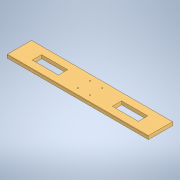
# Autodesk Inventor part: VerstaerkungHintenMitte
Saved by Autodesk Inventor 2020.3 (Build 243373010, 373A)
## iProperties
Created: 2021-02-13
Part Number: VerstaerkungHintenMitte
Material: Generisch
Document SubType Name: Modeling
Designer: Stefan
Density: 1 g/cm^3
Appearance: Fichte
Author: Stefan
Autodesk Inventor part; units mm, degrees
ref_plane "YZ Plane" through (0, 0, 0) normal (1, 0, 0) x (0, 1, 0)
ref_plane "XZ Plane" through (0, 0, 0) normal (0, 1, 0) x (-1, 0, 0)
ref_plane "XY Plane" through (0, 0, 0) normal (0, 0, 1) x (1, 0, 0)
sketch "Skizze1" plane through (0, 0, 0) normal (0, 1, 0) x (-1, 0, 0)
  line L0 (625.4144, 33.4967) -> (-184.5856, 33.4967)
  line L1 (-184.5856, 33.4967) -> (-184.5856, -108.5033)
  line L2 (-184.5856, -108.5033) -> (625.4144, -108.5033)
  line L3 (625.4144, -108.5033) -> (625.4144, 33.4967)
  line L4 (525.4144, -10.5033) -> (375.4144, -10.5033)
  line L5 (375.4144, -10.5033) -> (375.4144, -64.5033)
  line L6 (375.4144, -64.5033) -> (525.4144, -64.5033)
  line L7 (525.4144, -64.5033) -> (525.4144, -10.5033)
  line L8 (65.4144, -10.5033) -> (-84.5856, -10.5033)
  line L9 (-84.5856, -10.5033) -> (-84.5856, -64.5033)
  line L10 (-84.5856, -64.5033) -> (65.4144, -64.5033)
  line L11 (65.4144, -64.5033) -> (65.4144, -10.5033)
  circle A0 centre (255.4164, -2.5013) radius 3.1
  circle A1 centre (185.3764, -2.5013) radius 3.1
  circle A2 centre (255.4164, -72.5053) radius 3.1
  circle A3 centre (185.3764, -72.5053) radius 3.1
  point P0 (0, 0)
  dimension "d0" = 142
  dimension "d1" = 810
  dimension "d2" = 54
  dimension "d3" = 54
  dimension "d4" = 150
  dimension "d5" = 150
  dimension "d6" = 44
  dimension "d7" = 44
  dimension "d8" = 100
  dimension "d9" = 100
  dimension "d10" = 6.2
  dimension "d11" = 6.2
  dimension "d12" = 6.2
  dimension "d13" = 6.2
  dimension "d14" = 70.004
  dimension "d15" = 0
  dimension "d16" = 0
  dimension "d17" = 70.04
  dimension "d18" = 0
  dimension "d19" = 0
  dimension "d20" = 35.998
  dimension "d21" = 369.998
  constraints: 24 end point, 6 parallel, 4 centre point, 3 horizontal, 3 perpendicular
  measures "d0" distance of L0.end L1.end
  measures "d1" distance of L0.start L0.end
  measures "d2" distance of L6.end L4.start
  measures "d3" distance of L10.end L8.start
  measures "d4" distance of L5.end L6.end
  measures "d5" distance of L9.end L10.end
  measures "d6" distance between parallel lines of L0 L8
  measures "d7" distance between parallel lines of L0 L4
  measures "d8" distance between parallel lines of L3 L7
  measures "d9" distance between parallel lines of L1 L9
  measures "d10" diameter of A0
  measures "d11" diameter of A1
  measures "d12" diameter of A2
  measures "d13" diameter of A3
  measures "d14" distance of A3.centre A1.centre
  measures "d15" vertical distance of A1.centre A0.centre
  measures "d16" vertical distance of A3.centre A2.centre
  measures "d17" distance of A1.centre A0.centre
  measures "d18" horizontal distance of A0.centre A2.centre
  measures "d19" horizontal distance of A1.centre A3.centre
  measures "d20" distance from line of L0 A0.centre
  measures "d21" distance from line of L3 A0.centre
extrude "Extrusion1" add sketch "Skizze1" against normal blind 20
fillet "Rundung1" radius 2 4 edges at (-220.4144, -20, 33.4967) (-220.4144, 0, 33.4967) (-220.4144, -20, -108.5033) (-220.4144, 0, -108.5033)
